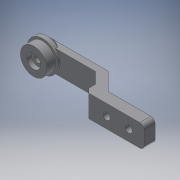
# Autodesk Inventor part: joint mag
Saved by Autodesk Inventor 2017 (Build 210142000, 142)
## iProperties
Created: 2021-02-27
Part Number: joint mag
Material: Generic
Document SubType Name: Modeling
Designer: paulg
Density: 1 g/cm^3
Appearance: Default
Author: paulg
Autodesk Inventor part; units mm, degrees
ref_plane "YZ Plane" through (0, 0, 0) normal (1, 0, 0) x (0, 1, 0)
ref_plane "XZ Plane" through (0, 0, 0) normal (0, 1, 0) x (-1, 0, 0)
ref_plane "XY Plane" through (0, 0, 0) normal (0, 0, 1) x (1, 0, 0)
sketch "Sketch1" plane through (0, 0, 0) normal (0, 0, 1) x (1, 0, 0)
  line L0 (0, 0) -> (0, 15)
  line L1 (0, 15) -> (23.6569, 15)
  line L2 (21, 12) -> (0, 12)
  line L3 (0, 12) -> (0, 15)
  line L4 (28, 0) -> (55, 0)
  line L5 (55, 0) -> (55, 5)
  line L6 (55, 5) -> (28, 5)
  line L7 (28, 5) -> (28, 0)
  line L8 (28, 5) -> (21, 12)
  line L9 (23.6569, 15) -> (33.6569, 5)
  dimension "d0" = 135
  dimension "d1" = 5
  dimension "d2" = 28
  dimension "d3" = 3
  dimension "d4" = 4
  dimension "d5" = 12
  dimension "d6" = 55
  constraints: 20 end point, 4 parallel, 2 horizontal, 2 point on line, 1 perpendicular, 1 vertical
  measures "d0" angle of L7 L8
  measures "d1" distance of L4.end L5.end
  measures "d2" distance from line of L4.start L0
  measures "d3" distance between parallel lines of L2 L1
  measures "d4" distance between parallel lines of L8 L9
  measures "d5" distance from line of L0.start L2
  measures "d6" distance of L4.end L0.start
extrude "Extrusion1" add sketch "Sketch1" along normal mid plane 10
sketch "Sketch3" plane through (33.6569, 5, 5) normal (0, 1, 0) x (1, 0, 0)
  line L0 (21.3431, 10) -> (21.3431, 0) projected
  line L1 (21.3431, 5) -> (-0.1629, 5) construction
  line L2 (-33.6569, 0) -> (-33.6569, 10) projected
  point P0 (-33.6569, 5)
  point P1 (14.3431, 5)
  point P2 (4.3431, 5)
  dimension "d9" = 10
  dimension "d18" = 38
  constraints: 2 end point, 2 point on line, 1 horizontal, 1 midpoint
  measures "d9" distance of point (14.343, 5) point (4.343, 5)
  measures "d18" distance from line of point (4.343, 5) L2
hole "Hole1" at (48, 5, 0) at (38, 5, 0) direction (0, -1, 0) diameter 3.2 end through all counterbore diameter 6.2 counterbore depth 2
chamfer "Chamfer1" distance 2 angle 45 1 edges at (28, 0, 0)
sketch "Sketch4" plane through (0, 15, 5) normal (0, 1, 0) x (1, 0, 0)
  circle A0 centre (0, 5) radius 6
  dimension "d22" = 12
  constraints: 1 centre point, 1 coincident
  measures "d22" diameter of A0
extrude "Extrusion2" add sketch "Sketch4" against normal up to surface (3 mm away)
sketch "Sketch5" plane through (21, 12, -5) normal (0, -1, 0) x (1, 0, 0)
  circle A0 centre (-21, 5) radius 6
  arc A1 (-17.6834, 10) -> (-17.6834, 0) centre (-21, 5) ccw projected
  constraints: 1 centre point, 1 coincident, 1 concentric
extrude "Extrusion3" add sketch "Sketch5" along normal blind 1
sketch "Sketch6" plane through (0, 11, 0) normal (0, -1, 0) x (1, 0, 0)
  circle A0 centre (0, 0) radius 5
  point P0 (0, 0)
  dimension "d27" = 10
  constraints: 1 centre point, 1 coincident
  measures "d27" diameter of A0
extrude "Extrusion4" add sketch "Sketch6" along normal blind 4
sketch "Sketch7" plane through (0, 7, 0) normal (0, -1, 0) x (1, 0, 0)
  circle A0 centre (0, 0) radius 3.1
  point P0 (0, 0)
  dimension "d30" = 6.2
  constraints: 1 centre point, 1 coincident
  measures "d30" diameter of A0
extrude "Extrusion5" cut sketch "Sketch7" against normal blind 2
sketch "Sketch8" plane through (23.6569, 15, 5) normal (0, 1, 0) x (1, 0, 0)
  circle A0 centre (-23.6569, 5) radius 1.6
  dimension "d33" = 3.2
  constraints: 1 centre point, 1 coincident
  measures "d33" diameter of A0
extrude "Extrusion6" cut sketch "Sketch8" against normal through all
chamfer "Chamfer2" [suppressed]
fillet "Fillet1" radius 2 2 edges at (55, 2.5, 5) (55, 2.5, -5)
body "Solid1"
